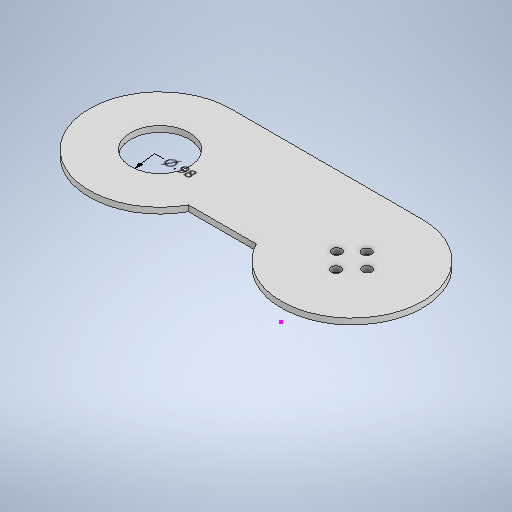
# Autodesk Inventor part: con_v8_d2_front
Saved by Autodesk Inventor 2025.4 (Build 294407000, 407)
## iProperties
Created: 2026-07-20
Part Number: con_v8_d2_front
Material: Generic
Document SubType Name: Modeling
Designer: Franchesca
Density: 1 g/cm^3
Appearance: Default
Author: Franchesca
Autodesk Inventor part; units mm, degrees
sketch "Sketch1" plane through (0, 0, 0) normal (0, 1, 0) x (-1, 0, 0)
  line L0 (30, 0) -> (-30, 0) construction
  arc A0 (-30, 32.5) -> (-30, -32.5) centre (-30, 0) ccw
  circle A1 centre (-30, 0) radius 32.5 construction
  circle A2 centre (-30, 0) radius 30 construction
  circle A3 centre (-30, -6.25) radius 2
  circle A4 centre (-30, 6.75) radius 2
  arc A5 (-15.4703, 26.2467) -> (-59.998, -0.3452) centre (-30, 0) ccw
  arc A6 (-3.6144, 14.2758) -> (-15.4703, 26.2467) centre (-30, 0) ccw
  arc A7 (-2.1644, 16.7758) -> (-30, 32.5) centre (-30, 0) ccw
  line L1 (-30, -6.25) -> (-30, 6.75) construction
  line L2 (-30, 0) -> (-36.5, 0) construction
  line L3 (-30, 0) -> (-23.5, 0) construction
  line L4 (-30, 0) -> (-23.5, 0) construction
  circle A8 centre (-23.5, 0) radius 2
  circle A9 centre (-36.5, 0) radius 2
  line L5 (-30, 0) -> (-30, -6.25) construction
  line L6 (-3.6144, 14.2758) -> (-3.6144, -14.2758) construction
  line L7 (-2.1644, 16.7758) -> (-2.1644, -16.7758) construction
  line L8 (-30, 32.5) -> (52.5439, 32.5) construction
  line L9 (-2.1644, 16.7758) -> (17.8356, 16.7758) construction
  line L10 (17.8356, 16.7758) -> (17.8356, -16.7758) construction
  line L11 (17.8356, -16.7758) -> (-2.1644, -16.7758) construction
  line L12 (-3.6144, -14.2758) -> (19.2856, -14.2758) construction
  line L13 (19.2856, -14.2758) -> (19.2856, 14.2758) construction
  line L14 (-3.6144, 14.2758) -> (19.2856, 14.2758) construction
  line L15 (0, 16.7758) -> (0, -16.7758) construction
  line L16 (2.5, 0) -> (2.5, 16.7758) construction
  line L17 (2.5, 0) -> (2.5, -16.7758) construction
  line L18 (19.2856, 0) -> (21.4496, 0) construction
  line L19 (21.4496, 0) -> (21.4496, 16.7758) construction
  line L20 (21.4496, 16.7758) -> (17.8356, 16.7758) construction
  line L21 (19.2856, 14.2758) -> (19.2856, 16.7758) construction
  line L22 (21.4496, 0) -> (21.4496, -16.7758) construction
  line L23 (21.4496, -16.7758) -> (17.8356, -16.7758) construction
  line L24 (19.2856, -14.2758) -> (19.2856, -16.7758) construction
  line L25 (21.4496, 0) -> (51.4496, 0) construction
  circle A10 centre (51.4496, 0) radius 30 construction
  circle A11 centre (51.4496, 0) radius 32.5 construction
  line L26 (19.2856, 14.2758) -> (25.064, 14.2758) construction
  line L27 (20.3676, 16.7758) -> (23.614, 16.7758) construction
  line L28 (17.3742, -16.7758) -> (23.614, -16.7758) construction
  line L29 (17.8356, -14.2758) -> (22.2529, -14.2758) construction
  line L30 (22.2529, -14.2758) -> (25.064, -14.2758) construction
  arc A12 (81.4496, 0) -> (51.4496, 30) centre (51.4496, 0) ccw
  arc A13 (51.4496, -30) -> (81.4496, 0) centre (51.4496, 0) ccw
  line L31 (51.4496, 30) -> (51.4496, -30) construction
  arc A14 (51.4496, 30) -> (25.064, 14.2758) centre (51.4496, 0) ccw
  line L32 (25.064, 14.2758) -> (-3.6144, 14.2758)
  line L33 (23.614, 16.7758) -> (-2.1644, 16.7758)
  arc A15 (51.4496, -32.5) -> (83.9496, 0) centre (51.4496, 0) ccw
  arc A16 (83.9496, 0) -> (51.4496, 32.5) centre (51.4496, 0) ccw
  arc A17 (51.4496, 32.5) -> (23.614, 16.7758) centre (51.4496, 0) ccw
  circle A18 centre (51.4496, 0) radius 12.5
  line L34 (51.4496, -32.5) -> (-30, -32.5)
  line L35 (51.4496, -30) -> (-30, -30)
  arc A19 (-59.998, -0.3452) -> (-30, -30) centre (-30, 0) ccw
  line L36 (8.3147, 14.2758) -> (8.3147, 30)
  point P0 (0, 0)
  point P1 (-30, 32.5)
  point P2 (-25, 0)
  point P3 (7.8356, 16.7758)
  dimension "d1" = 30
  dimension "d2" = 65
  dimension "d12" = 60
  dimension "d25" = 4
  dimension "d28" = 4
  dimension "d51" = 13
  dimension "d60" = 6.5
  dimension "d61" = 180
  dimension "d62" = 6.5
  dimension "d63" = 4
  dimension "d64" = 4
  dimension "d65" = 6.25
  dimension "d68" = 20
  dimension "d69" = 1.45
  dimension "d70" = 1.45
  dimension "d71" = 2.5
  dimension "d72" = 2.5
  dimension "d73" = 2.1644
  dimension "d74" = 2.164
  dimension "d75" = 30
  dimension "d76" = 60
  dimension "d77" = 65
  dimension "d78" = 60
  dimension "d79" = 25
  dimension "d116" = 81.4496
  dimension "d117" = 15.7241
  dimension "d118" = 2.5
  dimension "d119" = 2.5
  constraints: 76 end point, 42 point on circle, 20 centre point, 20 point on line, 10 perpendicular, 9 tangent, 8 concentric, 7 coincident, 7 vertical, 6 horizontal, 4 collinear, 3 midpoint, 1 parallel
  measures "d1" distance of point (0, 0) L0.end
  measures "d2" diameter of A0
  measures "d12" diameter of A2
  measures "d25" diameter of A3
  measures "d28" diameter of A4
  measures "d51" distance of L1.end L1.start
  measures "d60" distance of L2.start L2.end
  measures "d61" angle of L2 L3
  measures "d62" distance of L2.start L3.end
  measures "d63" diameter of A8
  measures "d64" diameter of A9
  measures "d65" distance of L2.start L1.start
  measures "d68" distance of L7.start L9.end
  measures "d69" distance between parallel lines of L6 L7
  measures "d70" distance between parallel lines of L10 L13
  measures "d71" distance between parallel lines of L11 L12
  measures "d72" distance from line of L14 point (7.836, 16.776)
  measures "d73" distance between parallel lines of L15 L7
  measures "d74" distance of L18.start L18.end
  measures "d75" distance of L18.end L25.end
  measures "d76" diameter of A10
  measures "d77" diameter of A11
  measures "d78" distance of L31.start L31.end
  measures "d79" diameter of A18
  measures "d116" distance of L31.end L35.end
  measures "d117" distance of L36.start L36.end
  measures "d118" distance between parallel lines of L35 L34
  measures "d119" radial gap between concentric circles of A10 A11
ref_plane "Work Plane1" through (0, -5, 0) normal (0, -1, 0) x (1, 0, 0)
ref_plane "Work Plane3" through (0, -35, 0) normal (0, -1, 0) x (1, 0, 0)
sketch "Sketch3" plane through (0, -35, 0) normal (0, -1, 0) x (1, 0, 0)
  point P0 (0, 0)
ref_plane "Work Plane4" through (0, -35, 0) normal (0, -1, 0) x (1, 0, 0)
extrude "Extrusion15" add sketch "Sketch1" along normal blind 2.5 contours L32 A14 A12 A13 L35 A19 A5 A6
body "Solid7"
